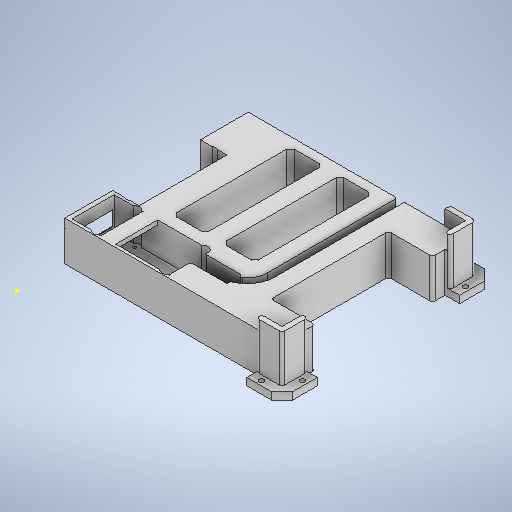
# Autodesk Inventor part: qrcode
Saved by Autodesk Inventor 2025.2 (Build 292293000, 293)
## iProperties
Created: 2025-11-10
Part Number: qrcode
Material: 일반
Document SubType Name: Modeling
Designer: RunGeun
Density: 1 g/cm^3
Appearance: 기본값
Author: RunGeun
Autodesk Inventor part; units mm, degrees
ref_plane "YZ Plane" through (0, 0, 0) normal (1, 0, 0) x (0, 1, 0)
ref_plane "XZ Plane" through (0, 0, 0) normal (0, 1, 0) x (-1, 0, 0)
ref_plane "XY Plane" through (0, 0, 0) normal (0, 0, 1) x (1, 0, 0)
sketch "스케치1" plane through (0, 0, 0) normal (0, 1, 0) x (-1, 0, 0)
  line L0 (0, 0) -> (260, 0)
  line L1 (260, 0) -> (260, -190)
  line L2 (260, -190) -> (0, -190)
  line L3 (0, -190) -> (0, 0)
  circle A0 centre (242, -18) radius 1.5
  circle A1 centre (242, -172) radius 1.5
  circle A2 centre (15, -175) radius 1.5
  circle A3 centre (13, -35) radius 1.5
  line L4 (242, -32.5) -> (112, -32.5)
  line L5 (112, -32.5) -> (112, -157.5)
  line L6 (112, -157.5) -> (242, -157.5)
  line L7 (242, -157.5) -> (242, -32.5)
  line L8 (242, -57.5) -> (258, -57.5)
  line L9 (258, -57.5) -> (258, -132.5)
  line L10 (258, -132.5) -> (242, -132.5)
  line L11 (242, -132.5) -> (242, -57.5)
  circle A4 centre (250, -67.5) radius 1.7
  circle A5 centre (250, -122.5) radius 1.7
  line L12 (18, -30) -> (3, -30)
  line L13 (3, -30) -> (3, -40)
  line L14 (3, -40) -> (18, -40)
  line L15 (18, -40) -> (18, -30)
  circle A6 centre (13, -155) radius 1.5
  line L16 (18, -150) -> (3, -150)
  line L17 (3, -150) -> (3, -160)
  line L18 (3, -160) -> (18, -160)
  line L19 (18, -160) -> (18, -150)
  line L20 (40, -172) -> (30, -172)
  circle A7 centre (35, -177) radius 1.5
  line L21 (40, -187) -> (40, -172)
  line L22 (30, -187) -> (40, -187)
  line L23 (30, -172) -> (30, -187)
  circle A8 centre (15, -15) radius 1.5
  circle A9 centre (35, -13) radius 1.5
  line L24 (40, -18) -> (40, -3)
  line L25 (40, -3) -> (30, -3)
  line L26 (30, -3) -> (30, -18)
  line L27 (30, -18) -> (40, -18)
  line L28 (230, -172) -> (220, -172)
  circle A10 centre (225, -177) radius 1.5
  line L29 (230, -187) -> (230, -172)
  line L30 (220, -187) -> (230, -187)
  line L31 (220, -172) -> (220, -187)
  line L32 (257, -169) -> (257, -159)
  circle A11 centre (247, -164) radius 1.5
  line L33 (242, -169) -> (257, -169)
  line L34 (242, -159) -> (242, -169)
  line L35 (257, -159) -> (242, -159)
  line L36 (257, -31) -> (257, -21)
  line L37 (242, -31) -> (257, -31)
  line L38 (257, -21) -> (242, -21)
  line L39 (242, -21) -> (242, -31)
  circle A12 centre (247, -26) radius 1.5
  circle A13 centre (225, -13) radius 1.5
  line L40 (220, -3) -> (220, -18)
  line L41 (220, -18) -> (230, -18)
  line L42 (230, -18) -> (230, -3)
  line L43 (230, -3) -> (220, -3)
  circle A14 centre (210, -15) radius 1.5
  circle A15 centre (110, -15) radius 1.5
  circle A16 centre (110, -175) radius 1.5
  circle A17 centre (210, -175) radius 1.5
  circle A18 centre (119, -25.5) radius 1.7
  circle A19 centre (105, -39.5) radius 1.7
  circle A20 centre (105, -150.5) radius 1.7
  circle A21 centre (119, -164.5) radius 1.7
  line L44 (126, -32.5) -> (102, -32.5)
  line L45 (102, -32.5) -> (102, -29.5)
  line L46 (109, -22.5) -> (126, -22.5)
  line L47 (126, -22.5) -> (126, -32.5)
  line L48 (102, -32.5) -> (112, -32.5)
  line L49 (112, -32.5) -> (112, -46.5)
  line L50 (112, -46.5) -> (102, -46.5)
  line L51 (102, -46.5) -> (102, -32.5)
  line L52 (102, -29.5) -> (109, -22.5)
  line L53 (126, -157.5) -> (102, -157.5)
  line L54 (102, -157.5) -> (102, -160.5)
  line L55 (109, -167.5) -> (126, -167.5)
  line L56 (126, -167.5) -> (126, -157.5)
  line L57 (102, -157.5) -> (112, -157.5)
  line L58 (112, -157.5) -> (112, -143.5)
  line L59 (112, -143.5) -> (102, -143.5)
  line L60 (102, -143.5) -> (102, -157.5)
  line L61 (102, -160.5) -> (109, -167.5)
  line L62 (260, -34.5) -> (191, -34.5)
  line L63 (191, -34.5) -> (191, -63.1)
  line L64 (191, -63.1) -> (260, -63.1)
  line L65 (260, -63.1) -> (260, -34.5)
  line L66 (260, -32.5) -> (189, -32.5)
  line L67 (189, -32.5) -> (189, -65.1)
  line L68 (189, -65.1) -> (260, -65.1)
  line L69 (260, -65.1) -> (260, -32.5)
  line L70 (260, -34.5) -> (257, -34.5)
  line L71 (257, -34.5) -> (257, -63.1)
  line L72 (257, -63.1) -> (260, -63.1)
  line L73 (260, -63.1) -> (260, -34.5)
  line L74 (257, -35.1) -> (260, -35.1)
  line L75 (260, -35.1) -> (260, -62.5)
  line L76 (260, -62.5) -> (257, -62.5)
  line L77 (257, -62.5) -> (257, -35.1)
  line L78 (191, -49.1) -> (166, -49.1)
  line L79 (166, -49.1) -> (166, -59.1)
  line L80 (166, -59.1) -> (191, -59.1)
  line L81 (191, -59.1) -> (191, -49.1)
  line L82 (158.6819, -157.5) -> (153.6819, -157.5)
  line L83 (153.6819, -157.5) -> (153.6819, -69.0321)
  line L84 (153.6819, -69.0321) -> (158.6819, -69.0321)
  line L85 (158.6819, -69.0321) -> (158.6819, -157.5)
  line L86 (166, -51.6) -> (166.6905, -51.6)
  line L87 (166.6905, -51.6) -> (166.6905, -56.6)
  line L88 (166.6905, -56.6) -> (166, -56.6)
  line L89 (166, -56.6) -> (166, -51.6)
  arc A22 (166, -56.6) -> (158.6819, -69.0321) centre (172.901, -69.0321) ccw
  arc A23 (166, -51.6) -> (153.6819, -69.0321) centre (172.1756, -69.0321) ccw
  line L90 (242, -157.5) -> (260, -157.5)
  line L91 (260, -157.5) -> (260, -32.5)
  line L92 (260, -32.5) -> (242, -32.5)
  line L93 (242, -32.5) -> (242, -157.5)
  line L94 (112, -55) -> (142, -55)
  line L95 (142, -55) -> (142, -135)
  line L96 (142, -135) -> (112, -135)
  line L97 (112, -135) -> (112, -55)
  line L98 (169.4017, -71.3) -> (191.4017, -71.3)
  line L99 (191.4017, -71.3) -> (191.4017, -151.3)
  line L100 (191.4017, -151.3) -> (169.4017, -151.3)
  line L101 (169.4017, -151.3) -> (169.4017, -71.3)
  line L102 (203.0959, -71.3) -> (225.0959, -71.3)
  line L103 (225.0959, -71.3) -> (225.0959, -151.3)
  line L104 (225.0959, -151.3) -> (203.0959, -151.3)
  line L105 (203.0959, -151.3) -> (203.0959, -71.3)
  circle A24 centre (194.45, -36.4) radius 1
  circle A25 centre (241, -36.4) radius 1
  circle A26 centre (241, -61.2) radius 1
  circle A27 centre (194.45, -61.2) radius 1
  line L106 (242, -157.5) -> (260, -157.5)
  line L107 (260, -157.5) -> (260, -132.5)
  line L108 (260, -132.5) -> (242, -132.5)
  line L109 (242, -132.5) -> (242, -157.5)
  line L110 (126, -32.5) -> (108.5, -32.5)
  line L111 (108.5, -32.5) -> (108.5, -29)
  line L112 (108.5, -29) -> (126, -29)
  line L113 (126, -29) -> (126, -32.5)
  line L114 (108.5, -32.5) -> (112, -32.5)
  line L115 (112, -32.5) -> (112, -46.5)
  line L116 (112, -46.5) -> (108.5, -46.5)
  line L117 (108.5, -46.5) -> (108.5, -32.5)
  line L118 (126, -157.5) -> (108.5, -157.5)
  line L119 (108.5, -157.5) -> (108.5, -161)
  line L120 (108.5, -161) -> (126, -161)
  line L121 (126, -161) -> (126, -157.5)
  line L122 (108.5, -157.5) -> (112, -157.5)
  line L123 (112, -157.5) -> (112, -143.5)
  line L124 (112, -143.5) -> (108.5, -143.5)
  line L125 (108.5, -143.5) -> (108.5, -157.5)
  line L126 (242, -132.5) -> (260, -132.5)
  line L127 (260, -132.5) -> (260, -124.9)
  line L128 (260, -124.9) -> (242, -124.9)
  line L129 (242, -124.9) -> (242, -132.5)
  point P0 (246.0334, -21.6633)
  point P1 (225, -187)
  point P2 (102, -22.5)
  point P3 (102, -167.5)
  point P4 (191, -54.1)
  point P5 (166.3452, -56.6)
  point P6 (214.0959, -151.3)
  point P7 (189, -49.1)
  point P8 (242, -65.1)
  point P9 (189, -59.1)
  point P10 (242, -34.5)
  point P11 (242, -63.1)
  point P12 (258, -65.1)
  dimension "d0" = 190
  dimension "d1" = 260
  dimension "d2" = 3
  dimension "d3" = 3
  dimension "d4" = 3
  dimension "d5" = 3
  dimension "d6" = 18
  dimension "d7" = 18
  dimension "d10" = 15
  dimension "d11" = 15
  dimension "d12" = 18
  dimension "d13" = 18
  dimension "d14" = 125
  dimension "d15" = 130
  dimension "d16" = 32.5
  dimension "d17" = 18
  dimension "d18" = 16
  dimension "d20" = 25
  dimension "d21" = 25
  dimension "d22" = 8
  dimension "d23" = 8
  dimension "d24" = 3.4
  dimension "d25" = 3.4
  dimension "d26" = 10
  dimension "d27" = 10
  dimension "d28" = 15
  dimension "d29" = 10
  dimension "d30" = 5
  dimension "d31" = 5
  dimension "d32" = 3
  dimension "d33" = 3
  dimension "d34" = 15
  dimension "d35" = 10
  dimension "d36" = 5
  dimension "d37" = 5
  dimension "d38" = 3
  dimension "d39" = 3
  dimension "d40" = 15
  dimension "d41" = 10
  dimension "d42" = 5
  dimension "d43" = 5
  dimension "d44" = 3
  dimension "d45" = 30
  dimension "d46" = 30
  dimension "d47" = 30
  dimension "d48" = 3
  dimension "d50" = 15
  dimension "d51" = 15
  dimension "d52" = 3
  dimension "d53" = 15
  dimension "d54" = 10
  dimension "d55" = 5
  dimension "d56" = 5
  dimension "d57" = 3
  dimension "d58" = 30
  dimension "d59" = 3
  dimension "d60" = 15
  dimension "d61" = 10
  dimension "d62" = 5
  dimension "d63" = 5
  dimension "d64" = 3
  dimension "d65" = 15
  dimension "d66" = 10
  dimension "d67" = 5
  constraints: 260 end point, 64 parallel, 32 perpendicular, 28 centre point, 28 horizontal, 18 point on line, 4 midpoint, 4 point on circle, 2 tangent
  measures "d0" distance of L0.end L1.end
  measures "d1" distance of L1.end L2.end
  measures "d2" diameter of A3
  measures "d3" diameter of A2
  measures "d4" diameter of A0
  measures "d5" diameter of A1
  measures "d6" distance from line of A0.centre L0
  measures "d7" distance from line of A0.centre L1
  measures "d10" distance from line of A2.centre L3
  measures "d11" distance from line of A2.centre L2
  measures "d12" distance from line of A1.centre L2
  measures "d13" distance from line of A1.centre L1
  measures "d14" distance of L6.end L4.start
  measures "d15" distance of L5.end L6.end
  measures "d16" distance between parallel lines of L4 L0
  measures "d17" distance between parallel lines of L7 L1
  measures "d18" distance of L9.end L10.end
  measures "d20" distance between parallel lines of L10 L6
  measures "d21" distance between parallel lines of L4 L8
  measures "d22" distance from line of A5.centre L7
  measures "d23" distance from line of A4.centre L11
  measures "d24" diameter of A4
  measures "d25" diameter of A5
  measures "d26" distance from line of A4.centre L8
  measures "d27" distance from line of A5.centre L10
  measures "d28" distance of L13.end L14.end
  measures "d29" distance of L14.end L12.start
  measures "d30" distance from line of A3.centre L14
  measures "d31" distance from line of A3.centre L15
  measures "d32" distance between parallel lines of L13 L3
  measures "d33" diameter of A6
  measures "d34" distance of L18.start L19.start
  measures "d35" distance of L19.start L19.end
  measures "d36" distance from line of A6.centre L18
  measures "d37" distance from line of A6.centre L19
  measures "d38" distance between parallel lines of L17 L3
  measures "d39" diameter of A7
  measures "d40" distance of L21.start L20.start
  measures "d41" distance of L20.start L20.end
  measures "d42" distance from line of A7.centre L21
  measures "d43" distance from line of A7.centre L20
  measures "d44" distance between parallel lines of L22 L2
  measures "d45" distance between parallel lines of L2 L18
  measures "d46" distance between parallel lines of L23 L3
  measures "d47" distance between parallel lines of L0 L12
  measures "d48" diameter of A8
  measures "d50" distance from line of A8.centre L3
  measures "d51" distance from line of A8.centre L0
  measures "d52" diameter of A9
  measures "d53" distance of L26.start L26.end
  measures "d54" distance of L26.end L27.end
  measures "d55" distance from line of A9.centre L26
  measures "d56" distance from line of A9.centre L27
  measures "d57" distance between parallel lines of L0 L25
  measures "d58" distance between parallel lines of L3 L26
  measures "d59" diameter of A10
  measures "d60" distance of L29.start L29.end
  measures "d61" distance of L29.end L28.end
  measures "d62" distance from line of A10.centre L29
  measures "d63" distance from line of A10.centre L28
  measures "d64" diameter of A11
  measures "d65" distance of L33.start L32.start
  measures "d66" distance of L32.start L32.end
  measures "d67" distance from line of A11.centre L33
extrude "돌출1" add sketch "스케치1" along normal blind 27 contours L1 L62 L7 L66 | L1 L74 L71 L62 | L7 L62 L63 L78 L67 L4 | L90 L7 L10 L108 L1 | L1 L76 L9 L8 L71 L74 | L67 L78 L79 A23 L83 L6 L5 L96 L95 L94 L4 | L108 L9 L128 L1 | L6 L85 A22 L79 L80 L67 L68 L7 | L1 L64 L9 L76 | L10 L7 L128 L9 | L1 L68 L9 L64 | L76 L71 L8 L9 | L9 L64 L71 L76 | L80 L63 L64 L7 L68 L67 | L9 L68 L7 L64
extrude "돌출2" add sketch "스케치1" along normal blind 5 contours L1 L62 L7 L66 | L1 L74 L71 L62 | L1 L76 L9 L8 L71 L74 | L71 L8 L7 L62 | L7 L64 L63 L62 | L1 L64 L9 L76 | L78 L63 L80 L67 | L67 L80 L79 L88 L87 L86 L78 | L6 L83 L84 L85 | L76 L71 L8 L9 | L9 L64 L71 L76 | L71 L64 L7 L8 | L84 A23 L79 A22 | L86 L87 L88 L79
extrude "돌출3" add sketch "스케치1" along normal blind 7 contours L10 L7 L128 L9 | L128 L7 L68 L9
sketch "스케치2" plane through (-260, 0, -65.1) normal (-1, 0, 0) x (0, 0, 1)
  point P0 (65.1, 0)
sketch "스케치3" plane through (-260, 0, -65.1) normal (-1, 0, 0) x (0, 0, 1)
  line L0 (2.8, 18.5) -> (29.8, 18.5)
  line L1 (29.8, 18.5) -> (29.8, 8.5)
  line L2 (29.8, 8.5) -> (2.8, 8.5)
  line L3 (2.8, 8.5) -> (2.8, 18.5)
  line L4 (0, 0) -> (32.6, 0) projected
  line L5 (0, 27) -> (32.6, 27) projected
  line L6 (32.6, 0) -> (32.6, 27) projected
  line L7 (0, 0) -> (0, 27) projected
  point P0 (65.1, 0)
  dimension "d174" = 8.5
  dimension "d178" = 10
  dimension "d179" = 27
  dimension "d180" = 2.8
  constraints: 8 end point, 2 parallel, 1 horizontal, 1 perpendicular
  measures "d174" distance between parallel lines of L4 L2
  measures "d178" distance between parallel lines of L2 L0
  measures "d179" distance of L0.start L0.end
  measures "d180" distance between parallel lines of L7 L3
extrude "돌출4" cut sketch "스케치3" against normal blind 27 contours L0 L1 L2 L3
chamfer "모따기1" distance 2.5 angle 45 4 edges at (-260, 8.5, -48.8) (-260, 13.5, -35.3) (-260, 18.5, -48.8) (-260, 13.5, -62.3)
chamfer "모따기2" distance 2.5 angle 45 8 edges at (-169.4017, 13.5, -151.3) (-191.4017, 13.5, -151.3) (-225.0959, 13.5, -151.3) (-203.0959, 13.5, -151.3) (-191.4017, 13.5, -71.3) (-169.4017, 13.5, -71.3) (-203.0959, 13.5, -71.3) (-225.0959, 13.5, -71.3)
extrude "돌출5" add sketch "스케치1" along normal blind 5 contours L112 L111 L44 L45 L52 L46 L47 | L117 L50 L51 L44 | L56 L55 L61 L54 L53 L119 L120 | L53 L60 L59 L125
extrude "돌출6" add sketch "스케치1" along normal blind 37 contours L4 L44 L111 L112 L47 | L5 L50 L117 L44 | L56 L120 L119 L53 L6 | L53 L125 L59 L5
fillet "모깎기1" radius 2 13 edges at (-142, 13.5, -55) (-112, 13.5, -55) (-112, 13.5, -135) (-142, 13.5, -135) (-112, 32, -46.5) (-126, 32, -32.5) (-108.5, 21, -46.5) (-126, 21, -29) (-108.5, 21, -29) (-108.5, 21, -161) (-126, 21, -161) (-112, 32, -143.5) (-108.5, 21, -143.5)
fillet "모깎기2" radius 1 9 edges at (-166, 16, -56.6) (-166, 16, -51.6) (-153.6819, 16, -157.5) (-158.6819, 16, -157.5) (-156.1819, 5, -157.5) (-191, 16, -59.1) (-191, 16, -49.1) (-166, 16, -59.1) (-166, 16, -49.1)
sketch "스케치4" plane through (0, 7, 0) normal (0, 1, 0) x (1, 0, 0)
  circle A0 centre (-250, 67.5) radius 1.7 projected
  circle A1 centre (-250, 67.5) radius 3
  circle A2 centre (-250, 122.5) radius 1.7 projected
  circle A3 centre (-250, 122.5) radius 3
  point P0 (0, 0)
  dimension "d199" = 6
  dimension "d200" = 6
  constraints: 2 centre point, 2 coincident
  measures "d199" diameter of A1
  measures "d200" diameter of A3
extrude "돌출7" cut sketch "스케치4" along normal blind 27
sketch "스케치5" plane through (-257, 27, -63.1) normal (0, 0, 1) x (1, 0, 0)
  line L0 (0, 0) -> (66, 0) projected
  line L1 (19.7078, 0) -> (29.7078, 0)
  line L2 (29.7078, 0) -> (29.7078, -3)
  line L3 (29.7078, -3) -> (19.7078, -3)
  line L4 (19.7078, -3) -> (19.7078, 0)
  point P0 (257, -27)
  dimension "d205" = 10
  dimension "d206" = 3
  constraints: 8 end point, 2 parallel, 1 horizontal, 1 perpendicular, 1 point on line
  measures "d205" distance of L2.end L3.end
  measures "d206" distance of L1.end L2.end
extrude "돌출8" add sketch "스케치5" along normal blind 29
sketch "스케치6" plane through (0, 5, 0) normal (0, 1, 0) x (1, 0, 0)
  circle A0 centre (-241, 61.2) radius 1 projected
  circle A1 centre (-241, 61.2) radius 3.4
  circle A2 centre (-241, 36.4) radius 1 projected
  circle A3 centre (-241, 36.4) radius 3.4
  circle A4 centre (-194.45, 61.2) radius 1 projected
  circle A5 centre (-194.45, 61.2) radius 3.4
  circle A6 centre (-194.45, 36.4) radius 1 projected
  circle A7 centre (-194.45, 36.4) radius 3.4
  point P0 (0, 0)
  dimension "d209" = 6.8
  dimension "d210" = 6.8
  dimension "d211" = 6.8
  dimension "d212" = 6.8
  constraints: 4 centre point, 4 coincident
  measures "d209" diameter of A1
  measures "d210" diameter of A3
  measures "d211" diameter of A7
  measures "d212" diameter of A5
extrude "돌출9" cut sketch "스케치6" along normal blind 29
equation "\"d3\" = d2"
equation "\"d4\" = d2"
equation "\"d5\" = d2"
equation "\"d7\" = d6"
equation "\"d11\" = d10"
equation "\"d12\" = d6"
equation "\"d13\" = d12"
equation "\"d22\" = d23"
equation "\"d25\" = d24"
equation "\"d31\" = d30"
equation "\"d37\" = d36"
equation "\"d43\" = d42"
